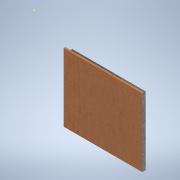
# Autodesk Inventor part: ДИ 00.00.08
Saved by Autodesk Inventor 2021.2 (Build 252289000, 289)
## iProperties
Created: 2021-10-12
Part Number: ДИ 00.00.08
Material: Типовые
Document SubType Name: Modeling
Designer: Surflay
Density: 1 g/cm^3
Appearance: По умолчанию
Author: Surflay
Autodesk Inventor part; units mm, degrees
ref_plane "YZ Plane" through (0, 0, 0) normal (1, 0, 0) x (0, 1, 0)
ref_plane "XZ Plane" through (0, 0, 0) normal (0, 1, 0) x (-1, 0, 0)
ref_plane "XY Plane" through (0, 0, 0) normal (0, 0, 1) x (1, 0, 0)
sketch "Эскиз1" plane through (0, 0, 0) normal (0, 0, 1) x (1, 0, 0)
  line L0 (123.5, -100.4305) -> (123.5, 102) projected
  arc A0 (93.5, -1) -> (113.5, -21) centre (113.5, -1) ccw projected
  line L1 (-123.5, 102) -> (-123.5, -102) projected
  line L2 (-123.5, -102) -> (123.5, -102) projected
  line L3 (123.5, -102) -> (123.5, -100.4305) projected
  line L4 (123.5, -100.4305) -> (123.5, 102) projected
  line L5 (123.5, 102) -> (-123.5, 102) projected
  line L6 (113.5, -21) -> (123.5, -21) projected
  line L7 (79.5, -18.0083) -> (79.5, -99) projected
  line L8 (123.5, -21) -> (39.5, -21)
  line L9 (39.5, -21) -> (39.5, -99)
  line L10 (39.5, -99) -> (123.5, -99)
  line L11 (123.5, -99) -> (123.5, -21)
  line L12 (121.5, -23) -> (41.5, -23)
  line L13 (41.5, -23) -> (41.5, -97)
  line L14 (41.5, -97) -> (121.5, -97)
  line L15 (121.5, -97) -> (121.5, -23)
  point P0 (0, 0)
  dimension "d0" = 3
  dimension "d1" = 2
  dimension "d2" = 2
  dimension "d3" = 2
  dimension "d4" = 2
  dimension "d5" = 80
  constraints: 16 end point, 4 parallel, 2 horizontal, 2 perpendicular
  measures "d0" distance between parallel lines of L2 L10
  measures "d1" distance between parallel lines of L13 L9
  measures "d2" distance between parallel lines of L10 L14
  measures "d3" distance between parallel lines of L0 L15
  measures "d4" distance between parallel lines of L8 L12
  measures "d5" distance between parallel lines of L15 L13
extrude "Выдавливание1" add sketch "Эскиз1" along normal blind 2 contours L10 L7 L14 L15 L12 L8 L6 L0 | L10 L9 L8 L7 L12 L13 L14
sketch "Эскиз2" plane through (0, 0, 2) normal (0, 0, 1) x (1, 0, 0)
  line L0 (39.5, -99) -> (123.5, -99) projected
  line L1 (33.5, -20.9806) -> (123.5, -20.9806)
  line L2 (123.5, -20.9806) -> (123.5, -99)
  line L3 (123.5, -99) -> (33.5, -99)
  line L4 (33.5, -99) -> (33.5, -20.9806)
  point P0 (0, 0)
  dimension "d8" = 78.0194
  dimension "d9" = 90
  constraints: 8 end point, 2 parallel, 1 horizontal, 1 perpendicular
  measures "d8" distance between parallel lines of L0 L1
  measures "d9" distance between parallel lines of L4 L2
extrude "Выдавливание2" add sketch "Эскиз2" along normal blind 2
sketch "Эскиз3" plane through (0, 0, 4) normal (0, 0, 1) x (1, 0, 0)
  point P0 (0, 0)
